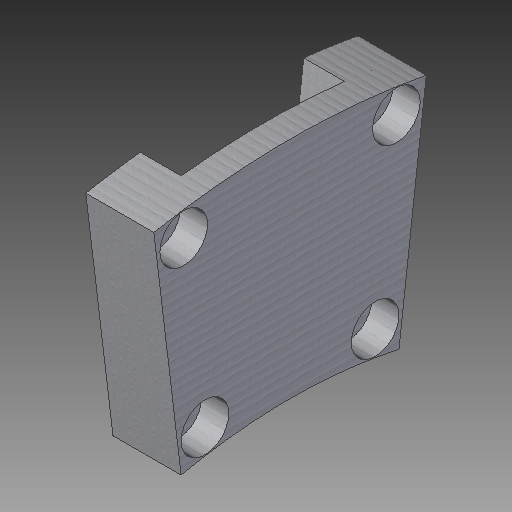
# Autodesk Inventor part: 32111_Lock Wedge Backing_V1
Saved by Autodesk Inventor 2020 (Build 240168000, 168)
## iProperties
Created: 2018-11-30
Part Number: 32111_Lock Wedge Backing_V1
Material: Acetal Resin, White
Document SubType Name: Modeling
Designer: MPI
Density: 1.425 g/cm^3
Appearance: Smooth - White
Mass: 1.29437 g
Surface Area: 11.0769 cm^2
Volume: 0.908329 cm^3
Author: MPI
Autodesk Inventor part; units mm, degrees
ref_plane "YZ Plane" through (0, 0, 0) normal (1, 0, 0) x (0, 1, 0)
ref_plane "XZ Plane" through (0, 0, 0) normal (0, 1, 0) x (-1, 0, 0)
ref_plane "XY Plane" through (0, 0, 0) normal (0, 0, 1) x (1, 0, 0)
sketch "Sketch1" plane through (0, 0, 0) normal (1, 0, 0) x (0, 1, 0)
  circle A0 centre (0, 0) radius 54
  circle A1 centre (0, 0) radius 37.5
  line L0 (37.5, 0) -> (54, 0)
  line L1 (53.066, -10) -> (36.6367, -8)
  line L2 (53.066, 10) -> (36.6367, 8)
  arc A2 (53.066, -10) -> (53.066, 10) centre (0, 0) ccw
  arc A3 (36.6367, -8) -> (36.6367, 8) centre (0, 0) ccw
  dimension "d0" = 108
  dimension "d1" = 75
  dimension "d2" = 10
  dimension "d3" = 0
  dimension "d4" = 8
  constraints: 10 point on circle, 6 end point, 4 centre point, 2 coincident, 2 symmetric about line, 1 horizontal
  measures "d0" diameter of A0
  measures "d1" diameter of A1
  measures "d2" vertical distance of L0.end L1.start
  measures "d3" distance from line of point (0, 0) L0
  measures "d4" vertical distance of L0.start L1.end
extrude "Extrusion1" add sketch "Sketch1" along normal blind 5 contours L0 A1 L2 A0 | A0 L1 A1 L0
sketch "Sketch2" plane through (0, 0, 0) normal (-1, 0, 0) x (0, 0, 1)
  arc A0 (10, 53.066) -> (-10, 53.066) centre (0, 0) ccw projected
  line L0 (-6, 53.6656) -> (-4, 37.2861)
  arc A1 (8, 36.6367) -> (-8, 36.6367) centre (0, 0) ccw projected
  line L1 (0, 54) -> (0, 37.5)
  line L2 (6, 53.6656) -> (4, 37.2861)
  arc A2 (6, 53.6656) -> (-6, 53.6656) centre (0, 0) ccw
  arc A3 (4, 37.2861) -> (-4, 37.2861) centre (0, 0) ccw
  point P0 (0, 0)
  dimension "d7" = 4
  dimension "d8" = 4
  constraints: 10 point on circle, 6 end point, 2 centre point, 2 symmetric about line
  measures "d7" horizontal distance of A0.end L0.start
  measures "d8" horizontal distance of A1.end L0.end
extrude "Extrusion2" cut sketch "Sketch2" against normal blind 3
sketch "Sketch3" plane through (5, 0, 0) normal (1, 0, 0) x (0, 0, -1)
  line L0 (-10, 53.066) -> (-8, 36.6367) projected
  circle A0 centre (0, 0) radius 52.2
  circle A1 centre (0, 0) radius 39.3
  circle A2 centre (-7.8083, 51.6127) radius 0.6
  circle A3 centre (-6.2486, 38.8001) radius 0.6
  line L1 (0, 54) -> (0, 37.3718)
  circle A4 centre (7.8083, 51.6127) radius 0.6
  circle A5 centre (6.2486, 38.8001) radius 0.6
  dimension "d15" = 104.4
  dimension "d16" = 78.6
  dimension "d17" = 1.2
  dimension "d18" = 1.2
  dimension "d19" = 2
  dimension "d20" = 2
  constraints: 4 centre point, 2 coincident, 2 end point, 2 symmetric about line, 1 vertical, 8 other
  measures "d17" diameter of A2
  measures "d18" diameter of A3
  measures "d19" distance from line of L0 A2.centre
  measures "d20" distance from line of L0 A3.centre
extrude "Extrusion3" cut sketch "Sketch3" against normal through all contours A2 A0 | A0 A2 | A3 A1 | A1 A3 | A4 A0 | A0 A4 | A5 A1 | A1 A5
sketch "Sketch4" plane through (5, 0, 0) normal (1, 0, 0) x (0, 0, -1)
  circle A0 centre (-7.8083, 51.6127) radius 0.6 projected
  circle A1 centre (-7.8083, 51.6127) radius 1.75
  circle A2 centre (7.8083, 51.6127) radius 0.6 projected
  circle A3 centre (7.8083, 51.6127) radius 1.75
  circle A4 centre (6.2486, 38.8001) radius 0.6 projected
  circle A5 centre (6.2486, 38.8001) radius 1.75
  circle A6 centre (-6.2486, 38.8001) radius 0.6 projected
  circle A7 centre (-6.2486, 38.8001) radius 1.75
  point P0 (0, 0)
  dimension "d23" = 3.5
  dimension "d24" = 3.5
  dimension "d25" = 3.5
  dimension "d26" = 3.5
  constraints: 4 centre point, 4 coincident
  measures "d23" diameter of A1
  measures "d24" diameter of A3
  measures "d25" diameter of A5
  measures "d26" diameter of A7
extrude "Extrusion4" cut sketch "Sketch4" against normal blind 2
body "Solid1"
